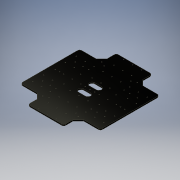
# Autodesk Inventor part: MountingPlate
Saved by Autodesk Inventor 2018 (Build 220112000, 112)
## iProperties
Created: 2018-11-01
Part Number: MountingPlate
Material: Generic
Document SubType Name: Modeling
Designer: anirudh
Density: 1 g/cm^3
Appearance: Gunmetal
Mass: 697.242 g
Surface Area: 2630.34 cm^2
Volume: 697.242 cm^3
Author: anirudh
Autodesk Inventor part; units mm, degrees
ref_plane "YZ Plane" through (0, 0, 0) normal (1, 0, 0) x (0, 1, 0)
ref_plane "XZ Plane" through (0, 0, 0) normal (0, 1, 0) x (-1, 0, 0)
ref_plane "XY Plane" through (0, 0, 0) normal (0, 0, 1) x (1, 0, 0)
sketch "Sketch1" plane through (0, 0, 0) normal (0, 1, 0) x (-1, 0, 0)
  line L0 (111.7346, 0) -> (259.1562, 0)
  line L1 (370.8908, -77.8256) -> (370.8908, -333.1718)
  line L2 (259.1562, -410.9974) -> (111.7346, -410.9974)
  line L3 (0, -333.1718) -> (0, -77.8256)
  line L4 (268.6812, -42.926) -> (294.1066, -68.3006)
  line L5 (294.1066, -342.6968) -> (268.6812, -368.0714)
  line L6 (102.2096, -42.926) -> (76.7842, -68.3006)
  line L7 (76.7842, -342.6968) -> (102.2096, -368.0714)
  line L8 (268.6812, -9.525) -> (268.6812, -42.926)
  line L9 (361.3658, -68.3006) -> (294.1066, -68.3006)
  line L10 (361.3658, -342.6968) -> (294.1066, -342.6968)
  line L11 (268.6812, -368.0714) -> (268.6812, -401.4724)
  line L12 (102.2096, -368.0714) -> (102.2096, -401.4724)
  line L13 (76.7842, -342.6968) -> (9.525, -342.6968)
  line L14 (76.7842, -68.3006) -> (9.525, -68.3006)
  line L15 (102.2096, -9.525) -> (102.2096, -42.926)
  circle A0 centre (185.4454, -7.62) radius 1.85
  circle A1 centre (227.0633, -7.62) radius 1.85
  circle A2 centre (143.8275, -7.62) radius 1.85
  circle A3 centre (227.0633, -403.3774) radius 1.85
  circle A4 centre (185.4454, -403.3774) radius 1.85
  circle A5 centre (143.8275, -403.3774) radius 1.85
  line L16 (361.3658, -68.3006) -> (346.3544, -68.3006)
  line L17 (9.525, -68.3006) -> (24.5364, -68.3006)
  circle A6 centre (346.3544, -205.4987) radius 1.85
  circle A7 centre (327.3044, -205.4987) radius 1.85
  circle A8 centre (308.2544, -205.4987) radius 1.85
  circle A9 centre (62.6364, -205.4987) radius 1.85
  circle A10 centre (43.5864, -205.4987) radius 1.85
  circle A11 centre (24.5364, -205.4987) radius 1.85
  circle A12 centre (228.092, -205.4987) radius 1.85
  circle A13 centre (142.7988, -205.5114) radius 1.85
  circle A14 centre (206.7814, -205.4987) radius 1.85
  circle A15 centre (185.4454, -205.4987) radius 1.85
  circle A16 centre (164.1602, -205.4987) radius 1.85
  circle A17 centre (102.9208, -129.286) radius 1.85
  circle A18 centre (102.9208, -281.7114) radius 1.85
  circle A19 centre (102.9208, -166.751) radius 1.85
  circle A20 centre (102.9208, -244.2464) radius 1.85
  circle A21 centre (102.9208, -205.5114) radius 1.85
  circle A22 centre (267.97, -166.751) radius 1.85
  circle A23 centre (267.97, -205.5114) radius 1.85
  circle A24 centre (267.97, -244.2464) radius 1.85
  circle A25 centre (267.97, -129.286) radius 1.85
  circle A26 centre (267.97, -281.7114) radius 1.85
  circle A27 centre (185.4454, -53.1114) radius 1.85
  circle A28 centre (185.4454, -103.9114) radius 1.85
  circle A29 centre (185.4454, -154.7114) radius 1.85
  circle A30 centre (185.4454, -256.286) radius 1.85
  circle A31 centre (185.4454, -307.086) radius 1.85
  circle A32 centre (185.4454, -357.886) radius 1.85
  circle A33 centre (226.7077, -53.1114) radius 1.85
  circle A34 centre (226.7077, -103.9114) radius 1.85
  circle A35 centre (226.7077, -154.7114) radius 1.85
  circle A36 centre (226.7077, -256.286) radius 1.85
  circle A37 centre (226.7077, -307.086) radius 1.85
  circle A38 centre (226.7077, -357.886) radius 1.85
  circle A39 centre (144.1831, -357.886) radius 1.85
  circle A40 centre (144.1831, -307.086) radius 1.85
  circle A41 centre (144.1831, -256.286) radius 1.85
  circle A42 centre (144.1831, -154.7114) radius 1.85
  circle A43 centre (144.1831, -103.9114) radius 1.85
  circle A44 centre (144.1831, -53.1114) radius 1.85
  circle A45 centre (350.5327, -103.9114) radius 1.85
  circle A46 centre (350.5327, -154.7114) radius 1.85
  circle A47 centre (350.5327, -256.286) radius 1.85
  circle A48 centre (350.5327, -307.086) radius 1.85
  circle A49 centre (309.2577, -103.9114) radius 1.85
  circle A50 centre (309.2577, -154.7114) radius 1.85
  circle A51 centre (309.2577, -256.286) radius 1.85
  circle A52 centre (309.2577, -307.086) radius 1.85
  circle A53 centre (294.1066, -129.286) radius 1.85
  circle A54 centre (294.1066, -281.7114) radius 1.85
  circle A55 centre (329.8952, -281.686) radius 1.85
  circle A56 centre (329.8952, -129.3114) radius 1.85
  circle A57 centre (61.6331, -103.9114) radius 1.85
  circle A58 centre (20.3581, -103.9114) radius 1.85
  circle A59 centre (61.6331, -154.7114) radius 1.85
  circle A60 centre (20.3581, -154.7114) radius 1.85
  circle A61 centre (61.6331, -256.286) radius 1.85
  circle A62 centre (20.3581, -256.286) radius 1.85
  circle A63 centre (61.6331, -307.086) radius 1.85
  circle A64 centre (20.3581, -307.086) radius 1.85
  circle A65 centre (40.9956, -129.3114) radius 1.85
  circle A66 centre (40.9956, -281.686) radius 1.85
  circle A67 centre (76.7842, -129.3114) radius 1.85
  circle A68 centre (76.7842, -281.7114) radius 1.85
  arc A69 (370.8908, -77.8256) -> (361.3658, -68.3006) centre (361.3658, -77.8256) ccw
  arc A70 (361.3658, -342.6968) -> (370.8908, -333.1718) centre (361.3658, -333.1718) ccw
  arc A71 (9.525, -68.3006) -> (0, -77.8256) centre (9.525, -77.8256) ccw
  arc A72 (0, -333.1718) -> (9.525, -342.6968) centre (9.525, -333.1718) ccw
  line L18 (268.6812, -23.9141) -> (268.6812, -9.525)
  arc A73 (268.6812, -9.525) -> (259.1562, 0) centre (259.1562, -9.525) ccw
  arc A74 (259.1562, -410.9974) -> (268.6812, -401.4724) centre (259.1562, -401.4724) ccw
  arc A75 (102.2096, -401.4724) -> (111.7346, -410.9974) centre (111.7346, -401.4724) ccw
  arc A76 (111.7346, 0) -> (102.2096, -9.525) centre (111.7346, -9.525) ccw
  circle A77 centre (267.97, -103.9114) radius 1.85
  circle A78 centre (267.97, -307.086) radius 1.85
  circle A79 centre (102.9208, -307.086) radius 1.85
  circle A80 centre (102.9208, -103.9114) radius 1.85
  circle A81 centre (247.3389, -77.8256) radius 1.85
  circle A82 centre (247.3389, -333.1718) radius 1.85
  circle A83 centre (123.5519, -333.1718) radius 1.85
  circle A84 centre (123.5519, -77.8256) radius 1.85
  circle A85 centre (268.6812, -68.3006) radius 1.85
  circle A86 centre (268.6812, -342.6968) radius 1.85
  circle A87 centre (102.2096, -342.6459) radius 1.85
  circle A88 centre (102.2096, -68.3006) radius 1.85
  point P0 (0, 0)
  constraints: 89 centre point, 38 end point, 16 point on circle, 7 perpendicular, 2 parallel, 2 point on line, 1 horizontal
extrude "Extrusion3" add sketch "Sketch1" along normal blind 5.588
sketch "Sketch3" plane through (0, 5.588, 0) normal (0, 1, 0) x (1, 0, 0)
  circle A0 centre (-226.7077, 256.286) radius 1.85 projected
  circle A1 centre (-228.092, 205.4987) radius 1.85 projected
  circle A2 centre (-226.7077, 154.7114) radius 1.85 projected
  circle A3 centre (-144.1831, 256.286) radius 1.85 projected
  circle A4 centre (-144.1831, 154.7114) radius 1.85 projected
  line L0 (-201.3077, 243.5924) -> (-169.5831, 243.5924)
  line L1 (-201.3077, 218.1924) -> (-169.5831, 218.1924)
  line L2 (-201.3077, 167.405) -> (-169.5831, 167.405)
  line L3 (-201.3077, 192.805) -> (-169.5831, 192.805)
  arc A5 (-169.5831, 167.405) -> (-169.5831, 192.805) centre (-169.5831, 180.105) ccw
  arc A6 (-201.3077, 192.805) -> (-201.3077, 167.405) centre (-201.3077, 180.105) ccw
  arc A7 (-169.5831, 218.1924) -> (-169.5831, 243.5924) centre (-169.5831, 230.8924) ccw
  arc A8 (-201.3077, 243.5924) -> (-201.3077, 218.1924) centre (-201.3077, 230.8924) ccw
  point P0 (0, 0)
  constraints: 8 end point, 8 point on circle, 4 centre point, 1 parallel
extrude "Extrusion4" cut sketch "Sketch3" against normal blind 25.4 contours L0 A7 L1 A8 | A6 L3 A5 L2
body "Solid3"
